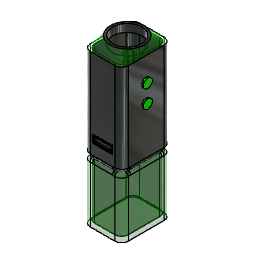
KeyHolder(DoorLocker) (Autodesk Fusion 360 design; units mm, degrees)
Autodesk Fusion 360 part; units mm, degrees
(part 1 of 8)
sketch "Sketch1" plane through (0, 0, 0) normal (0, 0, 1) x (1, 0, 0)
  line L0 (3, 0) -> (12, 0)
  line L1 (15, 3) -> (15, 17)
  line L2 (12, 20) -> (3, 20)
  line L3 (0, 17) -> (0, 3)
  line L4 (2, -1) -> (13, -1)
  line L5 (16, 2) -> (16, 18)
  line L6 (13, 21) -> (2, 21)
  line L7 (-1, 18) -> (-1, 2)
  arc A0 (12, 0) -> (15, 3) centre (12, 3) ccw
  arc A1 (13, -1) -> (16, 2) centre (13, 2) ccw
  arc A2 (-1, 2) -> (2, -1) centre (2, 2) ccw
  arc A3 (0, 3) -> (3, 0) centre (3, 3) ccw
  arc A4 (15, 17) -> (12, 20) centre (12, 17) ccw
  arc A5 (16, 18) -> (13, 21) centre (13, 18) ccw
  arc A6 (2, 21) -> (-1, 18) centre (2, 18) ccw
  arc A7 (3, 20) -> (0, 17) centre (3, 17) ccw
  point P0 (15, 0)
  point P1 (15, 20)
  dimension "d1" = 15
  dimension "d2" = 20
  dimension "d3" = 3
  dimension "d4" = 3
  constraint horizontal L0
  constraint perpendicular L0 L1
  constraint perpendicular L1 L2
  constraint perpendicular L0 L3
  constraint perpendicular L3 L4
  constraint perpendicular L4 L5
  constraint perpendicular L5 L6
  constraint perpendicular L4 L7
  constraint coincident P0 L0
  constraint coincident P0 L1
  constraint tangent L0 A0
  constraint tangent L1 A0
  constraint tangent L4 A1
  constraint tangent L5 A1
  constraint tangent L4 A2
  constraint tangent L7 A2
  constraint equal A1 A2
  constraint coincident origin L0
  constraint coincident origin L3
  constraint tangent L0 A3
  constraint tangent L3 A3
  constraint equal A1 A3
  constraint coincident P1 L1
  constraint coincident P1 L2
  constraint tangent L1 A4
  constraint tangent L2 A4
  constraint equal A1 A4
  constraint tangent L5 A5
  constraint tangent L6 A5
  constraint equal A1 A5
  constraint tangent L6 A6
  constraint tangent L7 A6
  constraint equal A1 A6
  constraint tangent L2 A7
  constraint tangent L3 A7
  constraint equal A1 A7
  measures "d1" distance of origin P0
  measures "d2" distance of P0 P1
  measures "d3" radius of A0
  measures "d4" radius of A1
extrude "Extrude1" add sketch "Sketch1" along normal blind 1.5 contours L0 L1 L2 L3 A0 A3 A4 A7 makes body 1
extrude "Extrude2" add sketch "Sketch1" along normal blind 26.5 bodies 1
fillet "Fillet1" radius 1.5 8 edges at (16, 10, 26.5) (15.1213, 20.1213, 26.5) (7.5, 21, 26.5) (-0.1213, 20.1213, 26.5) (-1, 10, 26.5) (-0.1213, -0.1213, 26.5) (7.5, -1, 26.5) (15.1213, -0.1213, 26.5) on bodies 1
ref_plane "WorkPlane1" through (7.5, 10, 27) normal (0, 0, 1) x (1, 0, 0)
sketch "Sketch2" plane through (0, 0, 27) normal (0, 0, 1) x (1, 0, 0)
  line L0 (0, 3) -> (0, 17)
  line L1 (3, 20) -> (12, 20)
  line L2 (15, 17) -> (15, 3)
  line L3 (12, 0) -> (3, 0)
  line L4 (-1, 18) -> (-1, 2)
  line L5 (2, -1) -> (13, -1)
  line L6 (16, 2) -> (16, 18)
  line L7 (13, 21) -> (2, 21)
  line L8 (6.5, 9) -> (6.5, 11)
  line L9 (6.5, 11) -> (8.5, 11)
  line L10 (8.5, 11) -> (8.5, 9)
  line L11 (8.5, 9) -> (6.5, 9)
  arc A0 (3, 20) -> (0, 17) centre (3, 17) ccw
  arc A1 (15, 17) -> (12, 20) centre (12, 17) ccw
  arc A2 (16, 18) -> (13, 21) centre (13, 18) ccw
  arc A3 (2, 21) -> (-1, 18) centre (2, 18) ccw
  arc A4 (0, 3) -> (3, 0) centre (3, 3) ccw
  arc A5 (-1, 2) -> (2, -1) centre (2, 2) ccw
  arc A6 (13, -1) -> (16, 2) centre (13, 2) ccw
  arc A7 (12, 0) -> (15, 3) centre (12, 3) ccw
  dimension "d12" = 3
  constraint vertical L0
  constraint perpendicular L0 L1
  constraint perpendicular L1 L2
  constraint perpendicular L0 L3
  constraint perpendicular L1 L4
  constraint perpendicular L4 L5
  constraint perpendicular L5 L6
  constraint perpendicular L4 L7
  constraint perpendicular L7 L8
  constraint perpendicular L8 L9
  constraint perpendicular L9 L10
  constraint perpendicular L8 L11
  constraint tangent L0 A0
  constraint tangent L1 A0
  constraint tangent L1 A1
  constraint tangent L2 A1
  constraint equal A0 A1
  constraint tangent L6 A2
  constraint tangent L7 A2
  constraint equal A0 A2
  constraint tangent L4 A3
  constraint tangent L7 A3
  constraint equal A0 A3
  constraint tangent L0 A4
  constraint tangent L3 A4
  constraint equal A0 A4
  constraint tangent L4 A5
  constraint tangent L5 A5
  constraint equal A0 A5
  constraint tangent L5 A6
  constraint tangent L6 A6
  constraint equal A0 A6
  constraint tangent L2 A7
  constraint tangent L3 A7
  constraint equal A0 A7
  measures "d12" radius of A0
extrude "Extrude3" add sketch "Sketch2" along normal blind 1.5 separate body contours L0 L1 L2 L3 A0 A1 A4 A7 makes body 2
extrude "Extrude4" add sketch "Sketch2" along normal blind 41.5 separate body contours L4 L5 L6 L7 A2 A3 A5 A6 makes body 3
fillet "Fillet2" radius 2 8 edges at (7.5, 21, 27) (-0.1213, 20.1213, 27) (-1, 10, 27) (-0.1213, -0.1213, 27) (7.5, -1, 27) (15.1213, -0.1213, 27) (16, 10, 27) (15.1213, 20.1213, 27) on bodies 3
sketch "Sketch3" plane through (16, 0, 0) normal (1, 0, 0) x (0, 1, 0)
  spline S0 degree 3 poles (3, 28.7321) (2.7604, 28.7321) (2.5207, 28.7593) (2.1893, 28.8136) (2.0946, 28.8309) (2, 28.8484) knots 2.269267 2.269267 2.269267 2.269267 2.341145 2.341145 2.37001 2.37001 2.37001 2.37001
  line L0 (3, 28.7321) -> (17, 28.7321)
  spline S1 degree 3 poles (18, 28.8484) (17.8364, 28.8181) (17.6727, 28.7887) (17.3396, 28.7452) (17.1697, 28.7321) (17, 28.7321) knots 2.168475 2.168475 2.168475 2.168475 2.218361 2.218361 2.269267 2.269267 2.269267 2.269267
  line L1 (18, 28.8484) -> (18, 68.5)
  line L2 (18, 68.5) -> (2, 68.5)
  line L3 (2, 68.5) -> (2, 28.8484)
  circle A0 centre (10, 58) radius 2
  circle A1 centre (10, 50) radius 2
  dimension "d19" = 4
  measures "d19" diameter of A1
extrude "Extrude1'" add sketch "Sketch3" along normal blind 0.7 separate body contours A0 | A1 makes body 4 at (16, 9.4492, 57.4257) makes body 5 at (16, 10.3333, 49.0296) in component "buttons"
ref_plane "WorkPlane2" through (7.5, 10, 72.5) normal (0, 0, 1) x (1, 0, 0)
sketch "Sketch4" plane through (0, 0, 72.5) normal (0, 0, 1) x (1, 0, 0)
  circle A0 centre (7.5, 10) radius 1.15
  circle A1 centre (7.5, 10) radius 1.35
  dimension "d23" = 2.3
  dimension "d24" = 2.7
  constraint concentric A0 A1
  measures "d23" diameter of A0
  measures "d24" diameter of A1
sketch "Sketch5" plane through (0, 0, 68.5) normal (0, 0, 1) x (-1, 0, 0)
  arc A0 (0, -3) -> (-3, 0) centre (-3, -3) ccw
  line L0 (0, -3) -> (0, -17)
  arc A1 (-3, -20) -> (0, -17) centre (-3, -17) ccw
  line L1 (-3, -20) -> (-12, -20)
  arc A2 (-15, -17) -> (-12, -20) centre (-12, -17) ccw
  line L2 (-15, -17) -> (-15, -3)
  arc A3 (-12, 0) -> (-15, -3) centre (-12, -3) ccw
  line L3 (-12, 0) -> (-3, 0)
  arc A4 (-13, 1) -> (-16, -2) centre (-13, -2) ccw
  line L4 (-16, -2) -> (-16, -18)
  arc A5 (-16, -18) -> (-13, -21) centre (-13, -18) ccw
  line L5 (-13, -21) -> (-2, -21)
  arc A6 (-2, -21) -> (1, -18) centre (-2, -18) ccw
  line L6 (1, -18) -> (1, -2)
  arc A7 (1, -2) -> (-2, 1) centre (-2, -2) ccw
  line L7 (-2, 1) -> (-13, 1)
  line L8 (-12, 0) -> (-3, 0)
  line L9 (0, -3) -> (0, -17)
  line L10 (-3, -20) -> (-12, -20)
  line L11 (-15, -17) -> (-15, -3)
  line L12 (-13, 1) -> (-2, 1)
  line L13 (1, -2) -> (1, -18)
  line L14 (-2, -21) -> (-13, -21)
  line L15 (-16, -18) -> (-16, -2)
  arc A8 (-12, 0) -> (-15, -3) centre (-12, -3) ccw
  arc A9 (0, -3) -> (-3, 0) centre (-3, -3) ccw
  arc A10 (-13, 1) -> (-16, -2) centre (-13, -2) ccw
  arc A11 (1, -2) -> (-2, 1) centre (-2, -2) ccw
  arc A12 (-15, -17) -> (-12, -20) centre (-12, -17) ccw
  arc A13 (-16, -18) -> (-13, -21) centre (-13, -18) ccw
  arc A14 (-2, -21) -> (1, -18) centre (-2, -18) ccw
  arc A15 (-3, -20) -> (0, -17) centre (-3, -17) ccw
  dimension "d25" = 3
  constraint horizontal L8
  constraint vertical L9
  constraint horizontal L10
  constraint vertical L11
  constraint horizontal L12
  constraint vertical L13
  constraint horizontal L14
  constraint vertical L15
  constraint tangent L8 A8
  constraint tangent L11 A8
  constraint tangent L8 A9
  constraint tangent L9 A9
  constraint equal A8 A9
  constraint tangent L12 A10
  constraint tangent L15 A10
  constraint equal A8 A10
  constraint tangent L12 A11
  constraint tangent L13 A11
  constraint equal A8 A11
  constraint tangent L10 A12
  constraint tangent L11 A12
  constraint equal A8 A12
  constraint tangent L14 A13
  constraint tangent L15 A13
  constraint equal A8 A13
  constraint tangent L13 A14
  constraint tangent L14 A14
  constraint equal A8 A14
  constraint tangent L9 A15
  constraint tangent L10 A15
  constraint equal A8 A15
  measures "d25" radius of A8
sketch "Sketch6" plane through (-1, 0, 0) normal (-1, 0, 0) x (0, -1, 0)
  line L0 (-2, 28.8484) -> (-2, 68.5)
  line L1 (-2, 68.5) -> (-18, 68.5)
  line L2 (-18, 68.5) -> (-18, 28.8484)
  spline S0 degree 3 poles (-2, 28.8484) (-2.2482, 28.8025) (-2.4977, 28.7587) (-2.8328, 28.7351) (-2.9165, 28.7321) (-3, 28.7321) knots 2.269626 2.269626 2.269626 2.269626 2.345342 2.345342 2.370384 2.370384 2.370384 2.370384
  spline S1 degree 3 poles (-17, 28.7321) (-17.0816, 28.7321) (-17.1635, 28.735) (-17.4992, 28.7581) (-17.75, 28.8021) (-18, 28.8484) knots 2.168462 2.168462 2.168462 2.168462 2.19293 2.19293 2.269201 2.269201 2.269201 2.269201
  line L3 (-17, 28.7321) -> (-3, 28.7321)
sketch "Sketch7" plane through (0, -1, 0) normal (0, -1, 0) x (1, 0, 0)
  line L0 (13, 28.8484) -> (13, 68.5)
  line L1 (13, 68.5) -> (2, 68.5)
  line L2 (2, 68.5) -> (2, 28.8484)
  line L3 (3, 37) -> (11.9661, 37)
  line L4 (11.9661, 37) -> (11.9661, 33.5)
  line L5 (11.9661, 33.5) -> (3, 33.5)
  line L6 (3, 33.5) -> (3, 37)
  line L7 (3.5, 36.5) -> (3.5, 34)
  line L8 (3.5, 34) -> (11.5, 34)
  line L9 (11.5, 34) -> (11.5, 36.5)
  line L10 (11.5, 36.5) -> (3.5, 36.5)
  line L11 (3.7, 36.3) -> (3.7, 34.2)
  line L12 (3.7, 34.2) -> (11.3, 34.2)
  line L13 (11.3, 34.2) -> (11.3, 36.3)
  line L14 (11.3, 36.3) -> (3.7, 36.3)
  spline S0 degree 3 poles (3, 28.7321) (2.7604, 28.7321) (2.5207, 28.7593) (2.1893, 28.8136) (2.0946, 28.8309) (2, 28.8484) knots 2.269267 2.269267 2.269267 2.269267 2.341145 2.341145 2.37001 2.37001 2.37001 2.37001
  line L15 (3, 28.7321) -> (12, 28.7321)
  spline S1 degree 3 poles (13, 28.8484) (12.7518, 28.8025) (12.5023, 28.7587) (12.1672, 28.7351) (12.0835, 28.7321) (12, 28.7321) knots 2.269626 2.269626 2.269626 2.269626 2.345342 2.345342 2.370384 2.370384 2.370384 2.370384
  dimension "d28" = 3.5
  constraint horizontal L3
  constraint vertical L4
  constraint horizontal L5
  constraint vertical L6
  constraint perpendicular L3 L7
  constraint perpendicular L7 L8
  constraint perpendicular L8 L9
  constraint perpendicular L7 L10
  constraint perpendicular L8 L11
  constraint perpendicular L11 L12
  constraint perpendicular L12 L13
  constraint perpendicular L11 L14
  measures "d28" distance of L3.start L5.end
extrude "Extrude6" cut sketch "Sketch7" against normal blind 0.75 contours L3 L4 L5 L6 bodies 3
extrude "Extrude7" cut sketch "Sketch7" against normal blind 0.75 contours L11 L12 L13 L14 bodies 3
sketch "Sketch8" plane through (-1, 10, 48.616) normal (-1, 0, 0) x (0, -1, 0)
  line L0 (-6, -12) -> (7, -12)
  line L1 (7, -12) -> (7, -17)
  line L2 (7, -17) -> (-6, -17)
  line L3 (-6, -17) -> (-6, -12)
  line L4 (-2.5, -12) -> (3.5, -12)
  line L5 (3.5, -12) -> (3.5, -11.5)
  line L6 (3.5, -11.5) -> (-2.5, -11.5)
  line L7 (-2.5, -11.5) -> (-2.5, -12)
  line L8 (-1, -11.5) -> (2, -11.5)
  line L9 (2, -11.5) -> (2, -11)
  line L10 (2, -11) -> (-1, -11)
  line L11 (-1, -11) -> (-1, -11.5)
  constraint horizontal L0
  constraint vertical L1
  constraint horizontal L2
  constraint vertical L3
  constraint horizontal L4
  constraint vertical L5
  constraint horizontal L6
  constraint vertical L7
  constraint coincident L0 L4.start
  constraint horizontal L8
  constraint vertical L9
  constraint horizontal L10
  constraint vertical L11
  constraint coincident L6 L8.start
extrude "Extrude8" cut sketch "Sketch8" against normal blind 0.05 contours L0 L1 L2 L3 L4 bodies 3
extrude "Extrude9" cut sketch "Sketch8" against normal blind 0.05 contours L6 L8 L9 L10 L11 bodies 3
extrude "Extrude10" cut sketch "Sketch8" against normal blind 0.5 contours L0 L4 L5 L6 L7 L8 bodies 3
sketch "Sketch9" plane through (16, 0, 0) normal (1, 0, 0) x (0, 1, 0)
  line L0 (2, 25.0318) -> (2, 0)
  line L1 (2, 0) -> (18, 0)
  line L2 (18, 0) -> (18, 25.0318)
  spline S0 degree 3 poles (2, 25.0318) (2.0838, 25.0384) (2.1673, 25.0452) (2.5002, 25.0709) (2.75, 25.0858) (3, 25.0858) knots 1.704045 1.704045 1.704045 1.704045 1.729213 1.729213 1.804213 1.804213 1.804213 1.804213
  spline S1 degree 3 poles (17, 25.0858) (17.043, 25.0858) (17.086, 25.0854) (17.4199, 25.0794) (17.71, 25.0544) (18, 25.0318) knots 1.704398 1.704398 1.704398 1.704398 1.7173 1.7173 1.804563 1.804563 1.804563 1.804563
  line L3 (17, 25.0858) -> (3, 25.0858)
ref_plane "WorkPlane3" through (7.5, 10, 72) normal (0, 0, 1) x (1, 0, 0)
sketch "Sketch10" plane through (0, 0, 72) normal (0, 0, 1) x (1, 0, 0)
  circle A0 centre (7.5, 10) radius 6.5
  dimension "d40" = 13
  measures "d40" diameter of A0
sketch "Sketch11" plane through (0, 0, 68.5) normal (0, 0, 1) x (-1, 0, 0)
  arc A0 (0, -3) -> (-3, 0) centre (-3, -3) ccw
  line L0 (0, -3) -> (0, -17)
  arc A1 (-3, -20) -> (0, -17) centre (-3, -17) ccw
  line L1 (-3, -20) -> (-12, -20)
  arc A2 (-15, -17) -> (-12, -20) centre (-12, -17) ccw
  line L2 (-15, -17) -> (-15, -3)
  arc A3 (-12, 0) -> (-15, -3) centre (-12, -3) ccw
  line L3 (-12, 0) -> (-3, 0)
  arc A4 (-13, 1) -> (-16, -2) centre (-13, -2) ccw
  line L4 (-16, -2) -> (-16, -18)
  arc A5 (-16, -18) -> (-13, -21) centre (-13, -18) ccw
  line L5 (-13, -21) -> (-2, -21)
  arc A6 (-2, -21) -> (1, -18) centre (-2, -18) ccw
  line L6 (1, -18) -> (1, -2)
  arc A7 (1, -2) -> (-2, 1) centre (-2, -2) ccw
  line L7 (-2, 1) -> (-13, 1)
  line L8 (-12, 0) -> (-3, 0)
  line L9 (0, -3) -> (0, -17)
  line L10 (-3, -20) -> (-12, -20)
  line L11 (-15, -17) -> (-15, -3)
  line L12 (-13, 1) -> (-2, 1)
  line L13 (1, -2) -> (1, -18)
  line L14 (-2, -21) -> (-13, -21)
  line L15 (-16, -18) -> (-16, -2)
  arc A8 (-12, 0) -> (-15, -3) centre (-12, -3) ccw
  arc A9 (-13, 1) -> (-16, -2) centre (-13, -2) ccw
  arc A10 (0, -3) -> (-3, 0) centre (-3, -3) ccw
  arc A11 (1, -2) -> (-2, 1) centre (-2, -2) ccw
  arc A12 (-3, -20) -> (0, -17) centre (-3, -17) ccw
  arc A13 (-2, -21) -> (1, -18) centre (-2, -18) ccw
  arc A14 (-16, -18) -> (-13, -21) centre (-13, -18) ccw
  arc A15 (-15, -17) -> (-12, -20) centre (-12, -17) ccw
  dimension "d41" = 3
  constraint horizontal L8
  constraint vertical L9
  constraint horizontal L10
  constraint vertical L11
  constraint horizontal L12
  constraint vertical L13
  constraint horizontal L14
  constraint vertical L15
  constraint tangent L8 A8
  constraint tangent L11 A8
  constraint tangent L12 A9
  constraint tangent L15 A9
  constraint equal A8 A9
  constraint tangent L8 A10
  constraint tangent L9 A10
  constraint equal A8 A10
  constraint tangent L12 A11
  constraint tangent L13 A11
  constraint equal A8 A11
  constraint tangent L9 A12
  constraint tangent L10 A12
  constraint equal A8 A12
  constraint tangent L13 A13
  constraint tangent L14 A13
  constraint equal A8 A13
  constraint tangent L14 A14
  constraint tangent L15 A14
  constraint equal A8 A14
  constraint tangent L10 A15
  constraint tangent L11 A15
  constraint equal A8 A15
  measures "d41" radius of A8
sketch "Sketch12" plane through (0, 0, 72) normal (0, 0, 1) x (1, 0, 0)
  circle A0 centre (7.5, 10) radius 7.5
  dimension "d42" = 15
  measures "d42" diameter of A0
loft "Loft2" add profiles "Sketch11", "Sketch12" section 1 section 2 bodies 3
extrude "Extrude11" cut sketch "Sketch10" against normal blind 3.5 bodies 3
sketch "Sketch13" plane through (0, 0, 27) normal (0, 0, -1) x (1, 0, 0)
  line L0 (8.5, -9) -> (8.5, -11)
  line L1 (8.5, -11) -> (6.5, -11)
  line L2 (6.5, -11) -> (6.5, -9)
  line L3 (6.5, -9) -> (8.5, -9)
  arc A0 (3, 0) -> (0, -3) centre (3, -3) ccw
  line L4 (0, -3) -> (0, -17)
  arc A1 (0, -17) -> (3, -20) centre (3, -17) ccw
  line L5 (3, -20) -> (12, -20)
  arc A2 (12, -20) -> (15, -17) centre (12, -17) ccw
  line L6 (15, -17) -> (15, -3)
  arc A3 (15, -3) -> (12, 0) centre (12, -3) ccw
  line L7 (12, 0) -> (3, 0)
  point P0 (7.5, -10)
sphere "SpherePrimitive1" add diameter 2 placed x (1, 0, 0) y (0, -1, 0) z (0, 0, -1) at (7.5, 10, 27) separate body makes body 6
sketch "Sketch15" plane through (-0.95, 0, 0) normal (-1, 0, 0) x (0, -1, 0)
  line L0 (-12.5, 36.616) -> (-16, 36.616)
  line L1 (-16, 36.616) -> (-16, 31.616)
  line L2 (-16, 31.616) -> (-3, 31.616)
  line L3 (-3, 31.616) -> (-3, 36.616)
  line L4 (-3, 36.616) -> (-6.5, 36.616)
  line L5 (-6.5, 36.616) -> (-12.5, 36.616)
sketch "Sketch16" plane through (-0.95, 0, 0) normal (-1, 0, 0) x (0, -1, 0)
copy_body "Body->Comp1" bodies 1 removing the originals makes body 7 in component "Dicoration part"
copy_body "Body->Comp2" bodies 3 removing the originals makes body 8 in component "body_function"
sketch "Sketch17" plane through (16, 0, 0) normal (1, 0, 0) x (0, 1, 0)
  spline S0 degree 3 poles (2, 25.0318) (2.0838, 25.0384) (2.1673, 25.0452) (2.5002, 25.0709) (2.75, 25.0858) (3, 25.0858) knots 1.704045 1.704045 1.704045 1.704045 1.729213 1.729213 1.804213 1.804213 1.804213 1.804213
  line L0 (2, 25.0318) -> (2, 0)
  line L1 (2, 0) -> (18, 0)
  line L2 (18, 0) -> (18, 25.0318)
  spline S1 degree 3 poles (17, 25.0858) (17.043, 25.0858) (17.086, 25.0854) (17.4199, 25.0794) (17.71, 25.0544) (18, 25.0318) knots 1.704398 1.704398 1.704398 1.704398 1.7173 1.7173 1.804563 1.804563 1.804563 1.804563
  line L3 (17, 25.0858) -> (3, 25.0858)
sketch "Sketch18" plane through (16, 0, 0) normal (1, 0, 0) x (0, 1, 0)
sketch "Sketch19" plane through (0, 0, 0) normal (0, 1, 0) x (1, 0, 0)
  spline S0 degree 3 poles (3.3781, -88.5364) (3.4032, -88.5157) (3.4336, -88.4768) (3.4432, -88.453) knots 0 0 0 0 1 1 1 1
  spline S1 degree 3 poles (3.4432, -88.453) (3.4479, -88.4298) (3.4271, -88.4449) (3.3902, -88.4922) knots 0 0 0 0 1 1 1 1
  spline S2 degree 3 poles (3.3902, -88.4922) (3.3555, -88.5367) (3.348, -88.5577) (3.3781, -88.5364) knots 0 0 0 0 1 1 1 1
  spline S3 degree 3 poles (3.8355, -88.0656) (3.859, -88.0526) (3.8758, -88.0254) (3.874, -88.0106) knots 0 0 0 0 1 1 1 1
  spline S4 degree 3 poles (3.874, -88.0106) (3.8743, -87.9929) (3.8529, -88.0031) (3.8318, -88.0359) knots 0 0 0 0 1 1 1 1
  spline S5 degree 3 poles (3.8318, -88.0359) (3.8079, -88.0664) (3.8098, -88.0813) (3.8355, -88.0656) knots 0 0 0 0 1 1 1 1
  spline S6 degree 3 poles (4.1304, -87.7454) (4.1415, -87.754) (4.2443, -87.7314) (4.3552, -87.6926) knots 0 0 0 0 1 1 1 1
  spline S7 degree 3 poles (4.3552, -87.6926) (4.4666, -87.6588) (4.5428, -87.6243) (4.5224, -87.6218) knots 0 0 0 0 1 1 1 1
  spline S8 degree 3 poles (4.5224, -87.6218) (4.4639, -87.6164) (4.1032, -87.7286) (4.1304, -87.7454) knots 0 0 0 0 1 1 1 1
  spline S9 degree 3 poles (4.1816, -87.8346) (4.1871, -87.8389) (4.2162, -87.8303) (4.2441, -87.8118) knots 0 0 0 0 1 1 1 1
  spline S10 degree 3 poles (4.2441, -87.8118) (4.2698, -87.7961) (4.2758, -87.7828) (4.2526, -87.7781) knots 0 0 0 0 1 1 1 1
  spline S11 degree 3 poles (4.2526, -87.7781) (4.2117, -87.7731) (4.1593, -87.8172) (4.1816, -87.8346) knots 0 0 0 0 1 1 1 1
  spline S12 degree 3 poles (4.5812, -87.6096) (4.5868, -87.6139) (4.6264, -87.6091) (4.6676, -87.5965) knots 0 0 0 0 1 1 1 1
  spline S13 degree 3 poles (4.6676, -87.5965) (4.7363, -87.583) (4.7357, -87.578) (4.663, -87.5794) knots 0 0 0 0 1 1 1 1
  spline S14 degree 3 poles (4.663, -87.5794) (4.5902, -87.5808) (4.559, -87.5922) (4.5812, -87.6096) knots 0 0 0 0 1 1 1 1
  line L0 (3.051, -89.8433) -> (3.0736, -89.946)
  line L1 (3.0736, -89.946) -> (3.0708, -89.8408)
  spline S15 degree 3 poles (3.0708, -89.8408) (3.0662, -89.7836) (3.0602, -89.7341) (3.0546, -89.7297) knots 0 0 0 0 1 1 1 1
  spline S16 degree 3 poles (3.0546, -89.7297) (3.0324, -89.7123) (3.0317, -89.7476) (3.051, -89.8433) knots 0 0 0 0 1 1 1 1
  spline S17 degree 3 poles (4.8285, -87.5566) (4.8808, -87.5527) (4.9276, -87.5444) (4.9341, -87.5361) knots 0 0 0 0 1 1 1 1
  spline S18 degree 3 poles (4.9341, -87.5361) (4.9406, -87.5278) (4.9026, -87.5249) (4.8503, -87.5288) knots 0 0 0 0 1 1 1 1
  spline S19 degree 3 poles (4.8503, -87.5288) (4.798, -87.5327) (4.7512, -87.541) (4.7447, -87.5493) knots 0 0 0 0 1 1 1 1
  spline S20 degree 3 poles (4.7447, -87.5493) (4.7382, -87.5576) (4.7762, -87.5605) (4.8285, -87.5566) knots 0 0 0 0 1 1 1 1
  spline S21 degree 3 poles (4.7636, -87.6626) (4.7692, -87.6669) (4.8088, -87.6621) (4.85, -87.6495) knots 0 0 0 0 1 1 1 1
  spline S22 degree 3 poles (4.85, -87.6495) (4.9187, -87.636) (4.9181, -87.631) (4.8454, -87.6324) knots 0 0 0 0 1 1 1 1
  spline S23 degree 3 poles (4.8454, -87.6324) (4.7727, -87.6338) (4.7414, -87.6452) (4.7636, -87.6626) knots 0 0 0 0 1 1 1 1
  spline S24 degree 3 poles (4.9713, -87.5114) (4.9768, -87.5158) (5.0164, -87.5109) (5.0576, -87.4983) knots 0 0 0 0 1 1 1 1
  spline S25 degree 3 poles (5.0576, -87.4983) (5.1263, -87.4848) (5.1257, -87.4799) (5.053, -87.4813) knots 0 0 0 0 1 1 1 1
  spline S26 degree 3 poles (5.053, -87.4813) (4.9803, -87.4827) (4.949, -87.494) (4.9713, -87.5114) knots 0 0 0 0 1 1 1 1
  spline S27 degree 3 poles (3.8321, -89.3075) (3.7254, -89.7479) (3.7206, -89.8113) (3.7283, -91.1022) knots 0 0 0 0 1 1 1 1
  spline S28 degree 3 poles (3.7283, -91.1022) (3.7288, -91.5771) (3.7215, -91.6609) (3.6605, -91.676) knots 0 0 0 0 1 1 1 1
  spline S29 degree 3 poles (3.6605, -91.676) (3.5995, -91.691) (3.5995, -91.691) (3.6574, -91.6914) knots 0 0 0 0 1 1 1 1
  spline S30 degree 3 poles (3.6574, -91.6914) (3.7152, -91.6919) (3.725, -91.9144) (3.726, -93.1507) knots 0 0 0 0 1 1 1 1
  spline S31 degree 3 poles (3.726, -93.1507) (3.7264, -93.9524) (3.7249, -94.6362) (3.7186, -94.6671) knots 0 0 0 0 1 1 1 1
  spline S32 degree 3 poles (3.7186, -94.6671) (3.7152, -94.7002) (3.6863, -94.7314) (3.6544, -94.7379) knots 0 0 0 0 1 1 1 1
  spline S33 degree 3 poles (3.6544, -94.7379) (3.6077, -94.7461) (3.5996, -94.7622) (3.6215, -94.7972) knots 0 0 0 0 1 1 1 1
  spline S34 degree 3 poles (3.6215, -94.7972) (3.6434, -94.8322) (3.6555, -94.8282) (3.6683, -94.7889) knots 0 0 0 0 1 1 1 1
  spline S35 degree 3 poles (3.6683, -94.7889) (3.7091, -94.6507) (3.7279, -94.8444) (3.7252, -95.4781) knots 0 0 0 0 1 1 1 1
  spline S36 degree 3 poles (3.7252, -95.4781) (3.7284, -95.8522) (3.7283, -96.5057) (3.7298, -96.9277) knots 0 0 0 0 1 1 1 1
  spline S37 degree 3 poles (3.7298, -96.9277) (3.7292, -97.3525) (3.7274, -97.7272) (3.7212, -97.7581) knots 0 0 0 0 1 1 1 1
  spline S38 degree 3 poles (3.7212, -97.7581) (3.7161, -97.799) (3.6883, -97.8175) (3.6304, -97.817) knots 0 0 0 0 1 1 1 1
  spline S39 degree 3 poles (3.6304, -97.817) (3.5527, -97.819) (3.5555, -97.8212) (3.6356, -97.839) knots 0 0 0 0 1 1 1 1
  spline S40 degree 3 poles (3.6356, -97.839) (3.687, -97.8478) (3.7268, -97.8655) (3.7253, -97.8732) knots 0 0 0 0 1 1 1 1
  spline S41 degree 3 poles (3.7253, -97.8732) (3.7374, -98.2588) (3.7215, -99.7461) (3.7106, -99.76) knots 0 0 0 0 1 1 1 1
  spline S42 degree 3 poles (3.7106, -99.76) (3.7019, -99.7711) (3.6295, -99.7951) (3.5503, -99.8048) knots 0 0 0 0 1 1 1 1
  line L2 (3.5503, -99.8048) -> (3.4079, -99.8323)
  line L3 (3.4079, -99.8323) -> (3.5549, -99.8218)
  spline S43 degree 3 poles (3.5549, -99.8218) (3.6319, -99.8149) (3.708, -99.8206) (3.7191, -99.8293) knots 0 0 0 0 1 1 1 1
  spline S44 degree 3 poles (3.7191, -99.8293) (3.7303, -99.838) (3.7892, -100.0318) (3.8491, -100.2532) knots 0 0 0 0 1 1 1 1
  spline S45 degree 3 poles (3.8491, -100.2532) (3.9068, -100.4773) (3.962, -100.6816) (3.97, -100.7058) knots 0 0 0 0 1 1 1 1
  spline S46 degree 3 poles (3.97, -100.7058) (4.0029, -100.7897) (4.618, -101.3777) (4.6647, -101.3694) knots 0 0 0 0 1 1 1 1
  spline S47 degree 3 poles (4.6647, -101.3694) (4.6895, -101.3664) (4.7075, -101.3491) (4.705, -101.3293) knots 0 0 0 0 1 1 1 1
  spline S48 degree 3 poles (4.705, -101.3293) (4.7026, -101.3095) (4.6816, -101.302) (4.6574, -101.31) knots 0 0 0 0 1 1 1 1
  spline S49 degree 3 poles (4.6574, -101.31) (4.6283, -101.3186) (4.5733, -101.2801) (4.4786, -101.1837) knots 0 0 0 0 1 1 1 1
  spline S50 degree 3 poles (4.4786, -101.1837) (4.406, -101.1046) (4.2745, -100.975) (4.1942, -100.8944) knots 0 0 0 0 1 1 1 1
  spline S51 degree 3 poles (4.1942, -100.8944) (4.0856, -100.7871) (4.0631, -100.7471) (4.1061, -100.7494) knots 0 0 0 0 1 1 1 1
  spline S52 degree 3 poles (4.1061, -100.7494) (4.1491, -100.7516) (4.1485, -100.7467) (4.0953, -100.7231) knots 0 0 0 0 1 1 1 1
  spline S53 degree 3 poles (4.0953, -100.7231) (4.0477, -100.7038) (4.007, -100.6183) (3.9542, -100.4338) knots 0 0 0 0 1 1 1 1
  spline S54 degree 3 poles (3.9542, -100.4338) (3.914, -100.2904) (3.8938, -100.1672) (3.913, -100.1599) knots 0 0 0 0 1 1 1 1
  spline S55 degree 3 poles (3.913, -100.1599) (3.9301, -100.1552) (3.9351, -100.1144) (3.9225, -100.0732) knots 0 0 0 0 1 1 1 1
  spline S56 degree 3 poles (3.9225, -100.0732) (3.909, -100.0045) (3.9041, -100.0051) (3.9077, -100.0751) knots 0 0 0 0 1 1 1 1
  spline S57 degree 3 poles (3.9077, -100.0751) (3.9044, -100.171) (3.8527, -100.1396) (3.8483, -100.0421) knots 0 0 0 0 1 1 1 1
  spline S58 degree 3 poles (3.8483, -100.0421) (3.8462, -100.0047) (3.8559, -99.9809) (3.867, -99.9896) knots 0 0 0 0 1 1 1 1
  spline S59 degree 3 poles (3.867, -99.9896) (3.8809, -100.0004) (3.8865, -99.9646) (3.8826, -99.9123) knots 0 0 0 0 1 1 1 1
  spline S60 degree 3 poles (3.8826, -99.9123) (3.8787, -99.86) (3.8572, -99.8073) (3.8356, -99.7949) knots 0 0 0 0 1 1 1 1
  spline S61 degree 3 poles (3.8356, -99.7949) (3.7796, -99.7691) (3.7792, -98.6809) (3.8346, -98.6615) knots 0 0 0 0 1 1 1 1
  spline S62 degree 3 poles (3.8346, -98.6615) (3.8609, -98.6508) (3.8625, -98.643) (3.8365, -98.6362) knots 0 0 0 0 1 1 1 1
  spline S63 degree 3 poles (3.8365, -98.6362) (3.8139, -98.6364) (3.7904, -98.5061) (3.7908, -98.3452) knots 0 0 0 0 1 1 1 1
  spline S64 degree 3 poles (3.7908, -98.3452) (3.7874, -98.0516) (3.8061, -97.9588) (3.8374, -98.0907) knots 0 0 0 0 1 1 1 1
  spline S65 degree 3 poles (3.8374, -98.0907) (3.8537, -98.1616) (3.8586, -98.161) (3.8551, -98.091) knots 0 0 0 0 1 1 1 1
  spline S66 degree 3 poles (3.8551, -98.091) (3.8573, -98.048) (3.8425, -98.0096) (3.8249, -98.0093) knots 0 0 0 0 1 1 1 1
  spline S67 degree 3 poles (3.8249, -98.0093) (3.8073, -98.0089) (3.7925, -97.9705) (3.7926, -97.9303) knots 0 0 0 0 1 1 1 1
  spline S68 degree 3 poles (3.7926, -97.9303) (3.7918, -97.8625) (3.794, -97.8598) (3.8282, -97.9134) knots 0 0 0 0 1 1 1 1
  spline S69 degree 3 poles (3.8282, -97.9134) (3.8597, -97.9648) (3.8646, -97.9642) (3.8623, -97.9042) knots 0 0 0 0 1 1 1 1
  spline S70 degree 3 poles (3.8623, -97.9042) (3.8602, -97.8667) (3.846, -97.8333) (3.8284, -97.8329) knots 0 0 0 0 1 1 1 1
  spline S71 degree 3 poles (3.8284, -97.8329) (3.7749, -97.8269) (3.7833, -96.2174) (3.8338, -96.1986) knots 0 0 0 0 1 1 1 1
  spline S72 degree 3 poles (3.8338, -96.1986) (3.8601, -96.1879) (3.8617, -96.1801) (3.8357, -96.1733) knots 0 0 0 0 1 1 1 1
  spline S73 degree 3 poles (3.8357, -96.1733) (3.8131, -96.1735) (3.7918, -96.0404) (3.7921, -95.8796) knots 0 0 0 0 1 1 1 1
  spline S74 degree 3 poles (3.7921, -95.8796) (3.7903, -95.5782) (3.8032, -95.4987) (3.8366, -95.6278) knots 0 0 0 0 1 1 1 1
  spline S75 degree 3 poles (3.8366, -95.6278) (3.8528, -95.6987) (3.8578, -95.6981) (3.8564, -95.6254) knots 0 0 0 0 1 1 1 1
  spline S76 degree 3 poles (3.8564, -95.6254) (3.8537, -95.583) (3.8445, -95.5489) (3.8297, -95.5507) knots 0 0 0 0 1 1 1 1
  spline S77 degree 3 poles (3.8297, -95.5507) (3.795, -95.555) (3.7672, -95.39) (3.7954, -95.3539) knots 0 0 0 0 1 1 1 1
  spline S78 degree 3 poles (3.7954, -95.3539) (3.8063, -95.34) (3.8242, -95.3629) (3.834, -95.4019) knots 0 0 0 0 1 1 1 1
  spline S79 degree 3 poles (3.834, -95.4019) (3.8502, -95.4728) (3.8552, -95.4722) (3.8538, -95.3995) knots 0 0 0 0 1 1 1 1
  spline S80 degree 3 poles (3.8538, -95.3995) (3.8511, -95.3571) (3.8419, -95.323) (3.8271, -95.3249) knots 0 0 0 0 1 1 1 1
  spline S81 degree 3 poles (3.8271, -95.3249) (3.7924, -95.3291) (3.7707, -95.2137) (3.7967, -95.1803) knots 0 0 0 0 1 1 1 1
  spline S82 degree 3 poles (3.7967, -95.1803) (3.8098, -95.1636) (3.8277, -95.1866) (3.8375, -95.2256) knots 0 0 0 0 1 1 1 1
  spline S83 degree 3 poles (3.8375, -95.2256) (3.8537, -95.2965) (3.8587, -95.2958) (3.8573, -95.2231) knots 0 0 0 0 1 1 1 1
  spline S84 degree 3 poles (3.8573, -95.2231) (3.8546, -95.1807) (3.8454, -95.1467) (3.8305, -95.1485) knots 0 0 0 0 1 1 1 1
  spline S85 degree 3 poles (3.8305, -95.1485) (3.7959, -95.1528) (3.7681, -94.9878) (3.7963, -94.9517) knots 0 0 0 0 1 1 1 1
  spline S86 degree 3 poles (3.7963, -94.9517) (3.8072, -94.9378) (3.8251, -94.9607) (3.8349, -94.9997) knots 0 0 0 0 1 1 1 1
  spline S87 degree 3 poles (3.8349, -94.9997) (3.8511, -95.0706) (3.8561, -95.07) (3.8525, -95) knots 0 0 0 0 1 1 1 1
  spline S88 degree 3 poles (3.8525, -95) (3.8548, -94.957) (3.84, -94.9186) (3.8224, -94.9183) knots 0 0 0 0 1 1 1 1
  spline S89 degree 3 poles (3.8224, -94.9183) (3.802, -94.9158) (3.7896, -94.8972) (3.7915, -94.8718) knots 0 0 0 0 1 1 1 1
  spline S90 degree 3 poles (3.7915, -94.8718) (3.7941, -94.8514) (3.8105, -94.8418) (3.8299, -94.857) knots 0 0 0 0 1 1 1 1
  spline S91 degree 3 poles (3.8299, -94.857) (3.8494, -94.8723) (3.8615, -94.8683) (3.8612, -94.8457) knots 0 0 0 0 1 1 1 1
  spline S92 degree 3 poles (3.8612, -94.8457) (3.8588, -94.8259) (3.8403, -94.798) (3.8236, -94.7849) knots 0 0 0 0 1 1 1 1
  spline S93 degree 3 poles (3.8236, -94.7849) (3.793, -94.7611) (3.772, -92.3585) (3.8018, -92.3146) knots 0 0 0 0 1 1 1 1
  spline S94 degree 3 poles (3.8018, -92.3146) (3.8098, -92.2985) (3.8237, -92.3094) (3.8345, -92.3357) knots 0 0 0 0 1 1 1 1
  spline S95 degree 3 poles (3.8345, -92.3357) (3.8431, -92.3648) (3.8502, -92.3614) (3.8565, -92.3305) knots 0 0 0 0 1 1 1 1
  spline S96 degree 3 poles (3.8565, -92.3305) (3.8578, -92.3002) (3.8476, -92.2788) (3.8328, -92.2806) knots 0 0 0 0 1 1 1 1
  spline S97 degree 3 poles (3.8328, -92.2806) (3.7981, -92.2849) (3.766, -92.1255) (3.7942, -92.0893) knots 0 0 0 0 1 1 1 1
  spline S98 degree 3 poles (3.7942, -92.0893) (3.8051, -92.0754) (3.8239, -92.0857) (3.8319, -92.1098) knots 0 0 0 0 1 1 1 1
  spline S99 degree 3 poles (3.8319, -92.1098) (3.8455, -92.1383) (3.8532, -92.1399) (3.8501, -92.1151) knots 0 0 0 0 1 1 1 1
  spline S100 degree 3 poles (3.8501, -92.1151) (3.8471, -92.0904) (3.8363, -92.064) (3.828, -92.0575) knots 0 0 0 0 1 1 1 1
  spline S101 degree 3 poles (3.828, -92.0575) (3.7919, -92.0293) (3.7738, -91.9435) (3.7955, -91.9157) knots 0 0 0 0 1 1 1 1
  spline S102 degree 3 poles (3.7955, -91.9157) (3.8085, -91.8991) (3.8274, -91.9093) (3.8354, -91.9335) knots 0 0 0 0 1 1 1 1
  spline S103 degree 3 poles (3.8354, -91.9335) (3.8489, -91.962) (3.8567, -91.9635) (3.8536, -91.9388) knots 0 0 0 0 1 1 1 1
  spline S104 degree 3 poles (3.8536, -91.9388) (3.8506, -91.914) (3.8343, -91.8833) (3.8176, -91.8703) knots 0 0 0 0 1 1 1 1
  spline S105 degree 3 poles (3.8176, -91.8703) (3.7981, -91.8551) (3.8044, -91.8242) (3.8316, -91.8007) knots 0 0 0 0 1 1 1 1
  spline S106 degree 3 poles (3.8316, -91.8007) (3.8589, -91.7773) (3.8587, -91.7547) (3.8299, -91.7456) knots 0 0 0 0 1 1 1 1
  spline S107 degree 3 poles (3.8299, -91.7456) (3.7774, -91.727) (3.7715, -90.3077) (3.8248, -90.2509) knots 0 0 0 0 1 1 1 1
  spline S108 degree 3 poles (3.8248, -90.2509) (3.8428, -90.2336) (3.8459, -90.2181) (3.8311, -90.22) knots 0 0 0 0 1 1 1 1
  spline S109 degree 3 poles (3.8311, -90.22) (3.7964, -90.2242) (3.7643, -90.0648) (3.7925, -90.0287) knots 0 0 0 0 1 1 1 1
  spline S110 degree 3 poles (3.7925, -90.0287) (3.8034, -90.0148) (3.8194, -90.0228) (3.8302, -90.0492) knots 0 0 0 0 1 1 1 1
  spline S111 degree 3 poles (3.8302, -90.0492) (3.841, -90.0755) (3.8459, -90.0749) (3.8522, -90.044) knots 0 0 0 0 1 1 1 1
  spline S112 degree 3 poles (3.8522, -90.044) (3.8541, -90.0186) (3.8412, -89.995) (3.8207, -89.9925) knots 0 0 0 0 1 1 1 1
  spline S113 degree 3 poles (3.8207, -89.9925) (3.7722, -89.9859) (3.7768, -89.8597) (3.8322, -89.8403) knots 0 0 0 0 1 1 1 1
  spline S114 degree 3 poles (3.8322, -89.8403) (3.8585, -89.8295) (3.8601, -89.8218) (3.8369, -89.8171) knots 0 0 0 0 1 1 1 1
  spline S115 degree 3 poles (3.8369, -89.8171) (3.7834, -89.8111) (3.9453, -89.1856) (4.0082, -89.1452) knots 0 0 0 0 1 1 1 1
  spline S116 degree 3 poles (4.0082, -89.1452) (4.0318, -89.1322) (4.0399, -89.1161) (4.0287, -89.1075) knots 0 0 0 0 1 1 1 1
  spline S117 degree 3 poles (4.0287, -89.1075) (3.9694, -89.0745) (3.9636, -89.0476) (4.0193, -89.0508) knots 0 0 0 0 1 1 1 1
  spline S118 degree 3 poles (4.0193, -89.0508) (4.0672, -89.0525) (4.0787, -89.0435) (4.0667, -89.0073) knots 0 0 0 0 1 1 1 1
  spline S119 degree 3 poles (4.0667, -89.0073) (4.0406, -88.9376) (4.4976, -88.4844) (4.5504, -88.5257) knots 0 0 0 0 1 1 1 1
  spline S120 degree 3 poles (4.5504, -88.5257) (4.5699, -88.5409) (4.5974, -88.54) (4.6105, -88.5233) knots 0 0 0 0 1 1 1 1
  spline S121 degree 3 poles (4.6105, -88.5233) (4.6213, -88.5094) (4.6118, -88.493) (4.5913, -88.4905) knots 0 0 0 0 1 1 1 1
  spline S122 degree 3 poles (4.5913, -88.4905) (4.5682, -88.4858) (4.5549, -88.4799) (4.5636, -88.4688) knots 0 0 0 0 1 1 1 1
  spline S123 degree 3 poles (4.5636, -88.4688) (4.5874, -88.4382) (5.2143, -88.2833) (5.2195, -88.3053) knots 0 0 0 0 1 1 1 1
  spline S124 degree 3 poles (5.2195, -88.3053) (5.2214, -88.3201) (5.1907, -88.3365) (5.1517, -88.3463) knots 0 0 0 0 1 1 1 1
  spline S125 degree 3 poles (5.1517, -88.3463) (5.1149, -88.3533) (5.0913, -88.3663) (5.0969, -88.3706) knots 0 0 0 0 1 1 1 1
  spline S126 degree 3 poles (5.0969, -88.3706) (5.1052, -88.3771) (5.1937, -88.3612) (5.2937, -88.3364) knots 0 0 0 0 1 1 1 1
  spline S127 degree 3 poles (5.2937, -88.3364) (5.3965, -88.3137) (5.4541, -88.2916) (5.4287, -88.2897) knots 0 0 0 0 1 1 1 1
  spline S128 degree 3 poles (5.4287, -88.2897) (5.3217, -88.2777) (5.427, -88.2346) (5.5504, -88.237) knots 0 0 0 0 1 1 1 1
  spline S129 degree 3 poles (5.5504, -88.237) (5.6238, -88.2406) (5.6869, -88.2228) (5.6888, -88.1974) knots 0 0 0 0 1 1 1 1
  spline S130 degree 3 poles (5.6888, -88.1974) (5.6929, -88.1692) (5.6979, -88.1686) (5.7114, -88.1971) knots 0 0 0 0 1 1 1 1
  spline S131 degree 3 poles (5.7114, -88.1971) (5.7302, -88.2476) (6.3094, -88.2569) (6.3154, -88.2034) knots 0 0 0 0 1 1 1 1
  spline S132 degree 3 poles (6.3154, -88.2034) (6.3157, -88.1858) (6.3541, -88.171) (6.3971, -88.1733) knots 0 0 0 0 1 1 1 1
  spline S133 degree 3 poles (6.3971, -88.1733) (6.4671, -88.1697) (6.4677, -88.1747) (6.3989, -88.1881) knots 0 0 0 0 1 1 1 1
  spline S134 degree 3 poles (6.3989, -88.1881) (6.3067, -88.2145) (6.3496, -88.257) (6.4453, -88.2377) knots 0 0 0 0 1 1 1 1
  spline S135 degree 3 poles (6.4453, -88.2377) (6.4821, -88.2307) (6.5028, -88.2156) (6.4917, -88.2069) knots 0 0 0 0 1 1 1 1
  spline S136 degree 3 poles (6.4917, -88.2069) (6.4806, -88.1982) (6.4992, -88.1859) (6.5311, -88.1794) knots 0 0 0 0 1 1 1 1
  spline S137 degree 3 poles (6.5311, -88.1794) (6.624, -88.158) (6.5975, -88.1059) (6.4978, -88.1131) knots 0 0 0 0 1 1 1 1
  spline S138 degree 3 poles (6.4978, -88.1131) (6.4483, -88.1192) (6.3255, -88.1217) (6.223, -88.1268) knots 0 0 0 0 1 1 1 1
  spline S139 degree 3 poles (6.223, -88.1268) (6.12, -88.1269) (6.037, -88.1471) (6.0345, -88.1675) knots 0 0 0 0 1 1 1 1
  spline S140 degree 3 poles (6.0345, -88.1675) (6.032, -88.1879) (6.0187, -88.182) (6.003, -88.1563) knots 0 0 0 0 1 1 1 1
  spline S141 degree 3 poles (6.003, -88.1563) (5.9873, -88.1306) (5.9424, -88.1135) (5.9078, -88.1177) knots 0 0 0 0 1 1 1 1
  spline S142 degree 3 poles (5.9078, -88.1177) (5.8681, -88.1226) (5.7475, -88.1223) (5.6312, -88.1165) knots 0 0 0 0 1 1 1 1
  spline S143 degree 3 poles (5.6312, -88.1165) (5.5198, -88.1101) (5.4201, -88.1173) (5.4115, -88.1284) knots 0 0 0 0 1 1 1 1
  spline S144 degree 3 poles (5.4115, -88.1284) (5.4006, -88.1423) (5.379, -88.1299) (5.3632, -88.1042) knots 0 0 0 0 1 1 1 1
  spline S145 degree 3 poles (5.3632, -88.1042) (5.338, -88.062) (5.3466, -88.0509) (5.4049, -88.0337) knots 0 0 0 0 1 1 1 1
  spline S146 degree 3 poles (5.4049, -88.0337) (5.4439, -88.0239) (5.4157, -88.0198) (5.3458, -88.0234) knots 0 0 0 0 1 1 1 1
  spline S147 degree 3 poles (5.3458, -88.0234) (5.2186, -88.0315) (5.144, -88.0582) (5.2569, -88.0569) knots 0 0 0 0 1 1 1 1
  spline S148 degree 3 poles (5.2569, -88.0569) (5.3021, -88.0564) (5.3144, -88.075) (5.3075, -88.1412) knots 0 0 0 0 1 1 1 1
  spline S149 degree 3 poles (5.3075, -88.1412) (5.303, -88.187) (5.2906, -88.2086) (5.2854, -88.1866) knots 0 0 0 0 1 1 1 1
  spline S150 degree 3 poles (5.2854, -88.1866) (5.2712, -88.1532) (5.0611, -88.1815) (4.875, -88.242) knots 0 0 0 0 1 1 1 1
  spline S151 degree 3 poles (4.875, -88.242) (4.8267, -88.258) (4.7218, -88.2835) (4.6481, -88.2975) knots 0 0 0 0 1 1 1 1
  spline S152 degree 3 poles (4.6481, -88.2975) (4.5305, -88.322) (4.466, -88.3702) (4.2601, -88.5764) knots 0 0 0 0 1 1 1 1
  spline S153 degree 3 poles (4.2601, -88.5764) (4.1212, -88.7141) (3.9931, -88.8379) (3.9745, -88.8502) knots 0 0 0 0 1 1 1 1
  spline S154 degree 3 poles (3.9745, -88.8502) (3.9538, -88.8653) (3.8911, -89.0716) (3.8321, -89.3075) knots 0 0 0 0 1 1 1 1
  spline S155 degree 3 poles (4.0764, -88.8402) (4.0782, -88.8551) (4.0614, -88.8823) (4.0379, -88.8952) knots 0 0 0 0 1 1 1 1
  spline S156 degree 3 poles (4.0379, -88.8952) (4.0121, -88.9109) (4.0103, -88.8961) (4.0342, -88.8655) knots 0 0 0 0 1 1 1 1
  spline S157 degree 3 poles (4.0342, -88.8655) (4.0553, -88.8328) (4.0767, -88.8226) (4.0764, -88.8402) knots 0 0 0 0 1 1 1 1
  spline S158 degree 3 poles (4.8532, -88.3101) (4.9259, -88.3087) (4.9265, -88.3136) (4.8578, -88.3271) knots 0 0 0 0 1 1 1 1
  spline S159 degree 3 poles (4.8578, -88.3271) (4.8166, -88.3397) (4.777, -88.3445) (4.7714, -88.3402) knots 0 0 0 0 1 1 1 1
  spline S160 degree 3 poles (4.7714, -88.3402) (4.7492, -88.3228) (4.7805, -88.3114) (4.8532, -88.3101) knots 0 0 0 0 1 1 1 1
  spline S161 degree 3 poles (5.0235, -88.264) (5.0962, -88.2626) (5.0968, -88.2676) (5.0281, -88.281) knots 0 0 0 0 1 1 1 1
  spline S162 degree 3 poles (5.0281, -88.281) (4.9869, -88.2936) (4.9473, -88.2985) (4.9417, -88.2942) knots 0 0 0 0 1 1 1 1
  spline S163 degree 3 poles (4.9417, -88.2942) (4.9195, -88.2768) (4.9508, -88.2654) (5.0235, -88.264) knots 0 0 0 0 1 1 1 1
  spline S164 degree 3 poles (5.3159, -88.2507) (5.3363, -88.2532) (5.348, -88.2669) (5.335, -88.2836) knots 0 0 0 0 1 1 1 1
  spline S165 degree 3 poles (5.335, -88.2836) (5.3241, -88.2975) (5.2929, -88.3088) (5.2724, -88.3063) knots 0 0 0 0 1 1 1 1
  spline S166 degree 3 poles (5.2724, -88.3063) (5.2493, -88.3016) (5.2403, -88.2902) (5.2533, -88.2735) knots 0 0 0 0 1 1 1 1
  spline S167 degree 3 poles (5.2533, -88.2735) (5.2642, -88.2596) (5.2927, -88.246) (5.3159, -88.2507) knots 0 0 0 0 1 1 1 1
  spline S168 degree 3 poles (3.8548, -99.8905) (3.8647, -99.9295) (3.8584, -99.9605) (3.8485, -99.9617) knots 0 0 0 0 1 1 1 1
  spline S169 degree 3 poles (3.8485, -99.9617) (3.8138, -99.9659) (3.7914, -99.8858) (3.8175, -99.8524) knots 0 0 0 0 1 1 1 1
  spline S170 degree 3 poles (3.8175, -99.8524) (3.8305, -99.8357) (3.8472, -99.8488) (3.8548, -99.8905) knots 0 0 0 0 1 1 1 1
  spline S171 degree 3 poles (4.4455, -88.2646) (4.4566, -88.2733) (4.5034, -88.265) (4.5538, -88.2463) knots 0 0 0 0 1 1 1 1
  spline S172 degree 3 poles (4.5538, -88.2463) (4.6405, -88.2155) (4.6405, -88.2155) (4.5381, -88.2206) knots 0 0 0 0 1 1 1 1
  spline S173 degree 3 poles (4.5381, -88.2206) (4.4335, -88.2284) (4.4121, -88.2385) (4.4455, -88.2646) knots 0 0 0 0 1 1 1 1
  spline S174 degree 3 poles (5.2455, -87.4526) (5.3232, -87.4506) (5.9337, -87.4485) (6.602, -87.4469) knots 0 0 0 0 1 1 1 1
  spline S175 degree 3 poles (6.602, -87.4469) (7.2731, -87.4474) (7.8279, -87.4422) (7.8344, -87.4338) knots 0 0 0 0 1 1 1 1
  spline S176 degree 3 poles (7.8344, -87.4338) (7.8409, -87.4255) (7.7599, -87.4204) (7.6519, -87.421) knots 0 0 0 0 1 1 1 1
  spline S177 degree 3 poles (7.6519, -87.421) (7.5467, -87.4239) (6.9659, -87.4223) (6.3604, -87.4238) knots 0 0 0 0 1 1 1 1
  spline S178 degree 3 poles (6.3604, -87.4238) (5.7521, -87.4231) (5.2255, -87.4325) (5.1837, -87.4401) knots 0 0 0 0 1 1 1 1
  spline S179 degree 3 poles (5.1837, -87.4401) (5.1425, -87.4527) (5.1707, -87.4568) (5.2455, -87.4526) knots 0 0 0 0 1 1 1 1
  spline S180 degree 3 poles (3.0531, -90.2702) (3.0694, -90.3411) (3.0743, -90.3405) (3.0729, -90.2678) knots 0 0 0 0 1 1 1 1
  spline S181 degree 3 poles (3.0729, -90.2678) (3.073, -90.2276) (3.0681, -90.188) (3.0626, -90.1836) knots 0 0 0 0 1 1 1 1
  spline S182 degree 3 poles (3.0626, -90.1836) (3.0403, -90.1663) (3.0369, -90.1994) (3.0531, -90.2702) knots 0 0 0 0 1 1 1 1
  spline S183 degree 3 poles (3.0496, -90.4466) (3.0659, -90.5175) (3.0708, -90.5169) (3.0694, -90.4442) knots 0 0 0 0 1 1 1 1
  spline S184 degree 3 poles (3.0694, -90.4442) (3.0695, -90.4039) (3.0647, -90.3643) (3.0591, -90.36) knots 0 0 0 0 1 1 1 1
  spline S185 degree 3 poles (3.0591, -90.36) (3.0369, -90.3426) (3.0334, -90.3757) (3.0496, -90.4466) knots 0 0 0 0 1 1 1 1
  spline S186 degree 3 poles (3.6248, -89.7276) (3.6387, -89.7384) (3.6635, -89.7354) (3.6744, -89.7215) knots 0 0 0 0 1 1 1 1
  spline S187 degree 3 poles (3.6744, -89.7215) (3.6874, -89.7048) (3.6822, -89.6828) (3.6683, -89.672) knots 0 0 0 0 1 1 1 1
  spline S188 degree 3 poles (3.6683, -89.672) (3.6516, -89.6589) (3.6318, -89.6614) (3.6188, -89.678) knots 0 0 0 0 1 1 1 1
  spline S189 degree 3 poles (3.6188, -89.678) (3.6079, -89.6919) (3.6082, -89.7145) (3.6248, -89.7276) knots 0 0 0 0 1 1 1 1
  spline S190 degree 3 poles (4.4809, -88.6146) (4.5045, -88.6017) (4.5212, -88.5745) (4.5194, -88.5596) knots 0 0 0 0 1 1 1 1
  spline S191 degree 3 poles (4.5194, -88.5596) (4.5198, -88.542) (4.4984, -88.5522) (4.4773, -88.5849) knots 0 0 0 0 1 1 1 1
  spline S192 degree 3 poles (4.4773, -88.5849) (4.4534, -88.6155) (4.4552, -88.6304) (4.4809, -88.6146) knots 0 0 0 0 1 1 1 1
  spline S193 degree 3 poles (3.0522, -90.6725) (3.0685, -90.7434) (3.0734, -90.7428) (3.072, -90.67) knots 0 0 0 0 1 1 1 1
  spline S194 degree 3 poles (3.072, -90.67) (3.0721, -90.6298) (3.0673, -90.5902) (3.0617, -90.5859) knots 0 0 0 0 1 1 1 1
  spline S195 degree 3 poles (3.0617, -90.5859) (3.0395, -90.5685) (3.036, -90.6016) (3.0522, -90.6725) knots 0 0 0 0 1 1 1 1
  spline S196 degree 3 poles (3.0548, -90.8983) (3.0711, -90.9692) (3.076, -90.9686) (3.0746, -90.8959) knots 0 0 0 0 1 1 1 1
  spline S197 degree 3 poles (3.0746, -90.8959) (3.0747, -90.8557) (3.0699, -90.8161) (3.0643, -90.8117) knots 0 0 0 0 1 1 1 1
  spline S198 degree 3 poles (3.0643, -90.8117) (3.0421, -90.7944) (3.0386, -90.8275) (3.0548, -90.8983) knots 0 0 0 0 1 1 1 1
  line L4 (3.0544, -91.0995) -> (3.0771, -91.2022)
  line L5 (3.0771, -91.2022) -> (3.0742, -91.097)
  spline S199 degree 3 poles (3.0742, -91.097) (3.0698, -90.9996) (3.0606, -90.9655) (3.0432, -90.9877) knots 0 0 0 0 1 1 1 1
  spline S200 degree 3 poles (3.0432, -90.9877) (3.0389, -90.9933) (3.0449, -91.0428) (3.0544, -91.0995) knots 0 0 0 0 1 1 1 1
  spline S201 degree 3 poles (5.5394, -88.0448) (5.545, -88.0492) (5.5846, -88.0443) (5.6258, -88.0317) knots 0 0 0 0 1 1 1 1
  spline S202 degree 3 poles (5.6258, -88.0317) (5.6945, -88.0183) (5.6939, -88.0133) (5.6212, -88.0147) knots 0 0 0 0 1 1 1 1
  spline S203 degree 3 poles (5.6212, -88.0147) (5.5485, -88.0161) (5.5172, -88.0275) (5.5394, -88.0448) knots 0 0 0 0 1 1 1 1
  line L6 (3.0542, -91.6097) -> (3.0705, -91.8238)
  line L7 (3.0705, -91.8238) -> (3.0719, -91.61)
  spline S204 degree 3 poles (3.0719, -91.61) (3.0692, -91.4244) (3.0619, -91.3649) (3.0445, -91.3872) knots 0 0 0 0 1 1 1 1
  spline S205 degree 3 poles (3.0445, -91.3872) (3.0401, -91.3927) (3.0446, -91.4902) (3.0542, -91.6097) knots 0 0 0 0 1 1 1 1
  spline S206 degree 3 poles (5.0461, -89.2263) (5.06, -89.2372) (5.0848, -89.2341) (5.0978, -89.2175) knots 0 0 0 0 1 1 1 1
  spline S207 degree 3 poles (5.0978, -89.2175) (5.1087, -89.2036) (5.0991, -89.1871) (5.0787, -89.1846) knots 0 0 0 0 1 1 1 1
  spline S208 degree 3 poles (5.0787, -89.1846) (5.0555, -89.1799) (5.0335, -89.1851) (5.027, -89.1935) knots 0 0 0 0 1 1 1 1
  spline S209 degree 3 poles (5.027, -89.1935) (5.0227, -89.199) (5.0294, -89.2133) (5.0461, -89.2263) knots 0 0 0 0 1 1 1 1
  spline S210 degree 3 poles (5.9416, -88.0457) (5.9472, -88.0501) (5.9868, -88.0452) (6.028, -88.0326) knots 0 0 0 0 1 1 1 1
  spline S211 degree 3 poles (6.028, -88.0326) (6.0967, -88.0191) (6.0961, -88.0142) (6.0234, -88.0156) knots 0 0 0 0 1 1 1 1
  spline S212 degree 3 poles (6.0234, -88.0156) (5.9507, -88.017) (5.9194, -88.0283) (5.9416, -88.0457) knots 0 0 0 0 1 1 1 1
  spline S213 degree 3 poles (3.0557, -91.9287) (3.0719, -91.9996) (3.0769, -91.999) (3.0755, -91.9262) knots 0 0 0 0 1 1 1 1
  spline S214 degree 3 poles (3.0755, -91.9262) (3.0756, -91.886) (3.0707, -91.8464) (3.0652, -91.8421) knots 0 0 0 0 1 1 1 1
  spline S215 degree 3 poles (3.0652, -91.8421) (3.0429, -91.8247) (3.0394, -91.8578) (3.0557, -91.9287) knots 0 0 0 0 1 1 1 1
  spline S216 degree 3 poles (5.5748, -88.7216) (5.5952, -88.7241) (5.6199, -88.7211) (5.6265, -88.7127) knots 0 0 0 0 1 1 1 1
  spline S217 degree 3 poles (5.6265, -88.7127) (5.6308, -88.7072) (5.6212, -88.6908) (5.6073, -88.6799) knots 0 0 0 0 1 1 1 1
  spline S218 degree 3 poles (5.6073, -88.6799) (5.5907, -88.6669) (5.5687, -88.6721) (5.5556, -88.6888) knots 0 0 0 0 1 1 1 1
  spline S219 degree 3 poles (5.5556, -88.6888) (5.5448, -88.7027) (5.5516, -88.7169) (5.5748, -88.7216) knots 0 0 0 0 1 1 1 1
  spline S220 degree 3 poles (3.0522, -92.105) (3.0684, -92.1759) (3.0734, -92.1753) (3.072, -92.1026) knots 0 0 0 0 1 1 1 1
  spline S221 degree 3 poles (3.072, -92.1026) (3.0721, -92.0624) (3.0672, -92.0228) (3.0617, -92.0184) knots 0 0 0 0 1 1 1 1
  spline S222 degree 3 poles (3.0617, -92.0184) (3.0394, -92.001) (3.036, -92.0341) (3.0522, -92.105) knots 0 0 0 0 1 1 1 1
  spline S223 degree 3 poles (6.1675, -88.0431) (6.1731, -88.0475) (6.2127, -88.0426) (6.2539, -88.03) knots 0 0 0 0 1 1 1 1
  spline S224 degree 3 poles (6.2539, -88.03) (6.3226, -88.0165) (6.322, -88.0116) (6.2493, -88.013) knots 0 0 0 0 1 1 1 1
  spline S225 degree 3 poles (6.2493, -88.013) (6.1766, -88.0144) (6.1453, -88.0257) (6.1675, -88.0431) knots 0 0 0 0 1 1 1 1
  spline S226 degree 3 poles (4.8124, -89.9839) (4.8263, -89.9947) (4.8511, -89.9917) (4.8641, -89.975) knots 0 0 0 0 1 1 1 1
  spline S227 degree 3 poles (4.8641, -89.975) (4.875, -89.9611) (4.8654, -89.9447) (4.845, -89.9422) knots 0 0 0 0 1 1 1 1
  spline S228 degree 3 poles (4.845, -89.9422) (4.8218, -89.9375) (4.7998, -89.9427) (4.7933, -89.951) knots 0 0 0 0 1 1 1 1
  spline S229 degree 3 poles (4.7933, -89.951) (4.789, -89.9566) (4.7957, -89.9708) (4.8124, -89.9839) knots 0 0 0 0 1 1 1 1
  line L8 (3.0544, -92.532) -> (3.077, -92.6348)
  line L9 (3.077, -92.6348) -> (3.0742, -92.5296)
  spline S230 degree 3 poles (3.0742, -92.5296) (3.0697, -92.4321) (3.0605, -92.3981) (3.0432, -92.4203) knots 0 0 0 0 1 1 1 1
  spline S231 degree 3 poles (3.0432, -92.4203) (3.0388, -92.4259) (3.0449, -92.4754) (3.0544, -92.532) knots 0 0 0 0 1 1 1 1
  spline S232 degree 3 poles (6.3074, -88.4658) (6.3213, -88.4766) (6.3643, -88.4789) (6.4055, -88.4663) knots 0 0 0 0 1 1 1 1
  spline S233 degree 3 poles (6.4055, -88.4663) (6.4742, -88.4528) (6.4714, -88.4507) (6.3891, -88.4356) knots 0 0 0 0 1 1 1 1
  spline S234 degree 3 poles (6.3891, -88.4356) (6.2991, -88.419) (6.2657, -88.4332) (6.3074, -88.4658) knots 0 0 0 0 1 1 1 1
  spline S235 degree 3 poles (3.0539, -92.7331) (3.0702, -92.804) (3.0751, -92.8034) (3.0737, -92.7307) knots 0 0 0 0 1 1 1 1
  spline S236 degree 3 poles (3.0737, -92.7307) (3.0738, -92.6905) (3.069, -92.6509) (3.0634, -92.6465) knots 0 0 0 0 1 1 1 1
  spline S237 degree 3 poles (3.0634, -92.6465) (3.0412, -92.6291) (3.0377, -92.6622) (3.0539, -92.7331) knots 0 0 0 0 1 1 1 1
  spline S238 degree 3 poles (6.5306, -88.2373) (6.5501, -88.2525) (6.5448, -88.2707) (6.5185, -88.2815) knots 0 0 0 0 1 1 1 1
  spline S239 degree 3 poles (6.5185, -88.2815) (6.4922, -88.2923) (6.4928, -88.2972) (6.5237, -88.3035) knots 0 0 0 0 1 1 1 1
  spline S240 degree 3 poles (6.5237, -88.3035) (6.5491, -88.3054) (6.5726, -88.2925) (6.5751, -88.272) knots 0 0 0 0 1 1 1 1
  spline S241 degree 3 poles (6.5751, -88.272) (6.5755, -88.2544) (6.6089, -88.2402) (6.6464, -88.2382) knots 0 0 0 0 1 1 1 1
  spline S242 degree 3 poles (6.6464, -88.2382) (6.6838, -88.2361) (6.7173, -88.2219) (6.7176, -88.2043) knots 0 0 0 0 1 1 1 1
  spline S243 degree 3 poles (6.7176, -88.2043) (6.718, -88.1866) (6.7563, -88.1719) (6.7994, -88.1741) knots 0 0 0 0 1 1 1 1
  spline S244 degree 3 poles (6.7994, -88.1741) (6.8693, -88.1706) (6.8699, -88.1755) (6.8012, -88.189) knots 0 0 0 0 1 1 1 1
  spline S245 degree 3 poles (6.8012, -88.189) (6.76, -88.2016) (6.7371, -88.2195) (6.7537, -88.2325) knots 0 0 0 0 1 1 1 1
  spline S246 degree 3 poles (6.7537, -88.2325) (6.7871, -88.2586) (6.9026, -88.2369) (6.8983, -88.2022) knots 0 0 0 0 1 1 1 1
  spline S247 degree 3 poles (6.8983, -88.2022) (6.8965, -88.1873) (6.9404, -88.1769) (6.9977, -88.1724) knots 0 0 0 0 1 1 1 1
  spline S248 degree 3 poles (6.9977, -88.1724) (7.0803, -88.1698) (7.088, -88.1714) (7.027, -88.1864) knots 0 0 0 0 1 1 1 1
  spline S249 degree 3 poles (7.027, -88.1864) (6.932, -88.2106) (6.9549, -88.233) (7.0978, -88.2506) knots 0 0 0 0 1 1 1 1
  spline S250 degree 3 poles (7.0978, -88.2506) (7.1667, -88.2597) (7.1277, -88.2695) (6.9913, -88.2838) knots 0 0 0 0 1 1 1 1